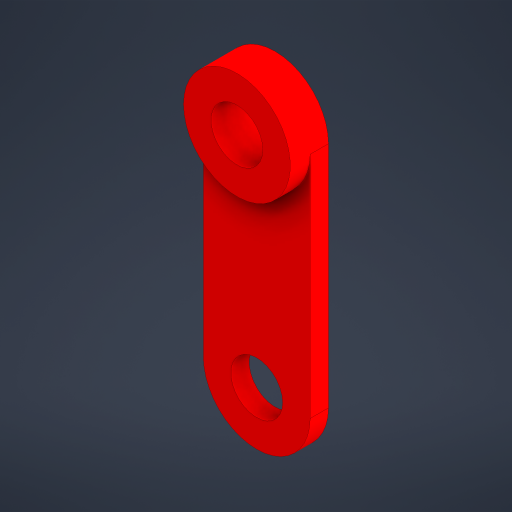
# Autodesk Inventor part: back qre flex holder
Saved by Autodesk Inventor 2024 (Build 280153000, 153)
## iProperties
Created: 2024-03-06
Part Number: back qre flex holder
Material: Všeobecné
Document SubType Name: Modeling
Designer: Simak
Density: 1 g/cm^3
Appearance: Výchozí
Author: Simak
Autodesk Inventor part; units mm, degrees
ref_plane "YZ Plane" through (0, 0, 0) normal (1, 0, 0) x (0, 1, 0)
ref_plane "XZ Plane" through (0, 0, 0) normal (0, 1, 0) x (-1, 0, 0)
ref_plane "XY Plane" through (0, 0, 0) normal (0, 0, 1) x (1, 0, 0)
sketch "Náčrt1" plane through (0, 0, 0) normal (0, 0, 1) x (1, 0, 0)
  line L0 (0, 7.5) -> (0, -7.5) construction
  line L1 (-3.5, 7.5) -> (-3.5, -7.5)
  line L2 (3.5, -7.5) -> (3.5, 7.5)
  arc A0 (3.5, 7.5) -> (-3.5, 7.5) centre (0, 7.5) ccw
  arc A1 (-3.5, -7.5) -> (3.5, -7.5) centre (0, -7.5) ccw
  circle A2 centre (0, 7.5) radius 1.7
  circle A3 centre (0, -7.5) radius 1.7
  circle A4 centre (0, 7.5) radius 3.5
  point P0 (0, 0)
  point P1 (0, 0)
  point P2 (3.5, 7.5)
  dimension "d0" = 15
  dimension "d1" = 3.5
  dimension "d2" = 3.4
  constraints: 8 end point, 5 centre point, 4 coincident, 4 point on circle, 4 tangent, 2 equal radius, 1 midpoint, 1 parallel, 1 vertical
  measures "d0" distance of L0.end L0.start
  measures "d1" radius of A0
  measures "d2" diameter of A2
extrude "Vysunutí1" add sketch "Náčrt1" along normal blind 1.2
extrude "Vysunutí2" add sketch "Náčrt1" along normal blind 2.5 contours A0 A4
